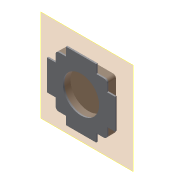
# Autodesk Inventor part: 30_Cube_counterplate_LEDmount
Saved by Autodesk Inventor 2019.4 (Build 234330000, 330)
## iProperties
Created: 2021-05-03
Part Number: 30_Cube_counterplate_LEDmount
Material: Generic
Document SubType Name: Modeling
Designer: diederichbenedict
Density: 1 g/cm^3
Appearance: Default
Author: diederichbenedict
Autodesk Inventor part; units mm, degrees
ref_plane "YZ Plane" through (0, 0, 0) normal (1, 0, 0) x (0, 1, 0)
ref_plane "XZ Plane" through (0, 0, 0) normal (0, 1, 0) x (-1, 0, 0)
ref_plane "XY Plane" through (0, 0, 0) normal (0, 0, 1) x (1, 0, 0)
ref_plane "Work Plane1" through (15.4052, 15.0652, 4.9) normal (0, 0, 1) x (0, 1, 0)
sketch "Sketch1" plane through (15.4052, 15.0652, 4.9) normal (0, 0, 1) x (0, 1, 0)
  circle A0 centre (5.7948, 15.4052) radius 2.5 projected
  circle A1 centre (-15.6052, -5.7948) radius 2.5 projected
  line L0 (-20.0856, 39.0762) -> (-20.0856, 40.2052) projected
  line L1 (-20.0856, 40.2052) -> (-38.2052, 40.2052) projected
  arc A2 (-38.2052, 40.2052) -> (-40.2052, 38.2052) centre (-38.2052, 38.2052) ccw projected
  line L2 (-40.2052, 20.2953) -> (-40.2052, 38.2052) projected
  line L3 (-40.2052, 20.2953) -> (-39.0783, 20.2953) projected
  arc A3 (-39.0783, 20.2953) -> (-38.6768, 20.6232) centre (-39.0783, 20.7051) ccw projected
  arc A4 (-34.5391, 20.2052) -> (-38.6768, 20.6232) centre (-36.6291, 20.2052) ccw projected
  line L4 (-34.5391, 20.2052) -> (-34.5391, 10.4067) projected
  arc A5 (-38.647, 9.8643) -> (-34.5391, 10.4067) centre (-36.6023, 10.2052) ccw projected
  line L5 (-38.647, 9.8643) -> (-38.6775, 9.9849) projected
  arc A6 (-38.6775, 9.9849) -> (-39.0762, 10.3249) centre (-39.083, 9.9131) ccw projected
  line L6 (-39.0762, 10.3249) -> (-40.2052, 10.3249) projected
  line L7 (-40.2052, -7.7948) -> (-40.2052, 10.3249) projected
  arc A7 (-40.2052, -7.7948) -> (-38.2052, -9.7948) centre (-38.2052, -7.7948) ccw projected
  line L8 (-38.2052, -9.7948) -> (-20.2052, -9.7948) projected
  line L9 (-20.2052, -9.7948) -> (-20.2052, -10.8453) projected
  arc A8 (-20.6052, -11.3352) -> (-20.2052, -10.8453) centre (-20.7052, -10.8453) ccw projected
  arc A9 (-20.6052, -11.3352) -> (-20.2052, -15.2948) centre (-20.2052, -13.2948) ccw projected
  line L10 (-20.2052, -15.2948) -> (-10.2052, -15.2948) projected
  arc A10 (-10.2052, -15.2948) -> (-9.8052, -11.3352) centre (-10.2052, -13.2948) ccw projected
  arc A11 (-10.2052, -10.8453) -> (-9.8052, -11.3352) centre (-9.7052, -10.8453) ccw projected
  line L11 (-10.2052, -10.8453) -> (-10.2052, -9.7948) projected
  line L12 (-10.2052, -9.7948) -> (7.7948, -9.7948) projected
  arc A12 (7.7948, -9.7948) -> (9.7948, -7.7948) centre (7.7948, -7.7948) ccw projected
  line L13 (9.7948, 10.2052) -> (9.7948, -7.7948) projected
  line L14 (9.7948, 10.2052) -> (10.8453, 10.2052) projected
  arc A13 (11.3352, 9.8052) -> (10.8453, 10.2052) centre (10.8453, 9.7052) ccw projected
  arc A14 (11.3352, 9.8052) -> (15.2948, 10.2052) centre (13.2948, 10.2052) ccw projected
  line L15 (15.2948, 10.2052) -> (15.2948, 20.2052) projected
  arc A15 (15.2948, 20.2052) -> (11.3352, 20.6052) centre (13.2948, 20.2052) ccw projected
  arc A16 (10.8453, 20.2052) -> (11.3352, 20.6052) centre (10.8453, 20.7052) ccw projected
  line L16 (10.8453, 20.2052) -> (9.7948, 20.2052) projected
  line L17 (9.7948, 38.2052) -> (9.7948, 20.2052) projected
  arc A17 (9.7948, 38.2052) -> (7.7948, 40.2052) centre (7.7948, 38.2052) ccw projected
  line L18 (7.7948, 40.2052) -> (-10.1151, 40.2052) projected
  line L19 (-10.1151, 40.2052) -> (-10.1151, 39.0783) projected
  arc A18 (-10.1151, 39.0783) -> (-9.7873, 38.6768) centre (-9.7054, 39.0783) ccw projected
  arc A19 (-10.2052, 34.5391) -> (-9.7873, 38.6768) centre (-10.2052, 36.6291) ccw projected
  line L20 (-10.2052, 34.5391) -> (-20.0038, 34.5391) projected
  arc A20 (-20.5462, 38.647) -> (-20.0038, 34.5391) centre (-20.2052, 36.6023) ccw projected
  line L21 (-20.5462, 38.647) -> (-20.4256, 38.6775) projected
  arc A21 (-20.4256, 38.6775) -> (-20.0856, 39.0762) centre (-20.4974, 39.083) ccw projected
  line L22 (-0.2052, 32.2052) -> (-30.2052, 32.2052) projected
  arc A22 (1.7948, 30.2052) -> (-0.2052, 32.2052) centre (-0.2052, 30.2052) ccw projected
  line L23 (1.7948, 30.2052) -> (1.7948, 0.2052) projected
  arc A23 (-0.2052, -1.7948) -> (1.7948, 0.2052) centre (-0.2052, 0.2052) ccw projected
  line L24 (-0.2052, -1.7948) -> (-30.2052, -1.7948) projected
  arc A24 (-32.2052, 0.2052) -> (-30.2052, -1.7948) centre (-30.2052, 0.2052) ccw projected
  line L25 (-32.2052, 0.2052) -> (-32.2052, 30.2052) projected
  arc A25 (-30.2052, 32.2052) -> (-32.2052, 30.2052) centre (-30.2052, 30.2052) ccw projected
  circle A26 centre (-35.2052, 35.2052) radius 2.425 projected
  circle A27 centre (-29.7052, 36.0052) radius 2.65 projected
  circle A28 centre (-36.0052, 29.7052) radius 2.65 projected
  circle A29 centre (-35.2052, -4.7948) radius 2.425 projected
  circle A30 centre (-29.7052, -5.5948) radius 2.65 projected
  circle A31 centre (-36.0052, 0.7052) radius 2.65 projected
  circle A32 centre (4.7948, 35.2052) radius 2.425 projected
  circle A33 centre (-0.7052, 36.0052) radius 2.65 projected
  circle A34 centre (5.5948, 29.7052) radius 2.65 projected
  circle A35 centre (5.5948, 0.7052) radius 2.65 projected
  circle A36 centre (-0.7052, -5.5948) radius 2.65 projected
  circle A37 centre (4.7948, -4.7948) radius 2.425 projected
  point P0 (-15.0652, 15.4052)
extrude "Extrusion1" add sketch "Sketch1" against normal blind 5 draft -1 contours A22 L23 A23 L24 A24 L25 A25 L22
sketch "Sketch2" plane through (15.4052, 15.0652, 4.9) normal (0, 0, 1) x (1, 0, 0)
  circle A0 centre (-26.2552, -7.0652) radius 3 projected
  circle A1 centre (-26.2552, -23.0652) radius 3 projected
  circle A2 centre (-4.2552, -15.0652) radius 1.6 projected
  line L0 (-50.1952, -15.0652) -> (19.3848, -15.0652)
  circle A3 centre (-15.4052, -15.0652) radius 12
  dimension "d4" = 24
  constraints: 2 end point, 1 centre point, 1 coincident, 1 horizontal, 2 other
  measures "d4" diameter of A3
extrude "Extrusion2" cut sketch "Sketch2" against normal blind 4 contours A0 A3 | A0 A3 A2 L0 | A3 L0 A2 | L0 A2 A3 A1 | L0 A3 A2 | A1 A3 picked at (-24.6691, -8.292) picked at (-4.1694, -14.672) picked at (-4.1694, -15.4584) picked at (-24.6691, -21.8384)
sketch "Sketch4" plane through (15.4052, 15.0652, 4.9) normal (0, 0, 1) x (1, 0, 0)
  circle A0 centre (-15.4052, -15.0652) radius 12 construction
  line L0 (-32.2052, -0.2052) -> (-32.2052, -30.2052) construction
  arc A1 (-32.2052, -30.2052) -> (-30.2052, -32.2052) centre (-30.2052, -30.2052) ccw construction
  line L1 (-30.2052, -32.2052) -> (-0.2052, -32.2052) construction
  arc A2 (-0.2052, -32.2052) -> (1.7948, -30.2052) centre (-0.2052, -30.2052) ccw construction
  line L2 (1.7948, -30.2052) -> (1.7948, -0.2052) construction
  arc A3 (1.7948, -0.2052) -> (-0.2052, 1.7948) centre (-0.2052, -0.2052) ccw construction
  line L3 (-0.2052, 1.7948) -> (-30.2052, 1.7948) construction
  arc A4 (-30.2052, 1.7948) -> (-32.2052, -0.2052) centre (-30.2052, -0.2052) ccw construction
  line L4 (-37.9052, -25.0652) -> (7.0948, -25.0652) construction
  line L5 (7.0948, -25.0652) -> (7.0948, -5.0652) construction
  line L6 (7.0948, -5.0652) -> (-37.9052, -5.0652) construction
  line L7 (-37.9052, -5.0652) -> (-37.9052, -25.0652) construction
  line L8 (-37.9052, -25.0652) -> (7.0948, -5.0652) construction
  line L9 (7.0948, -25.0652) -> (-37.9052, -5.0652) construction
  line L10 (-25.4052, 7.4348) -> (-5.4052, 7.4348) construction
  line L11 (-5.4052, 7.4348) -> (-5.4052, -37.5652) construction
  line L12 (-5.4052, -37.5652) -> (-25.4052, -37.5652) construction
  line L13 (-25.4052, -37.5652) -> (-25.4052, 7.4348) construction
  line L14 (-25.4052, 7.4348) -> (-5.4052, -37.5652) construction
  line L15 (-5.4052, 7.4348) -> (-25.4052, -37.5652) construction
  line L16 (1.7075, -30.2052) -> (1.7075, -0.2052) construction
  line L17 (-30.2052, -32.2052) -> (-0.2052, -32.2052) construction
  line L18 (-32.118, -0.2052) -> (-32.118, -30.2052) construction
  line L19 (-0.2052, 1.7948) -> (-30.2052, 1.7948) construction
  line L20 (7.0948, -5.0652) -> (1.7075, -5.0652)
  line L21 (1.7075, -5.0652) -> (1.7075, -25.0652)
  line L22 (1.7075, -25.0652) -> (7.0948, -25.0652)
  line L23 (7.0948, -25.0652) -> (7.0948, -5.0652)
  line L24 (-5.4052, -37.5652) -> (-25.4052, -37.5652)
  line L25 (-25.4052, -37.5652) -> (-25.4052, -32.2052)
  line L26 (-25.4052, -32.2052) -> (-5.4052, -32.2052)
  line L27 (-5.4052, -32.2052) -> (-5.4052, -37.5652)
  line L28 (-32.2052, -25.0652) -> (-37.9052, -25.0652)
  line L29 (-37.9052, -25.0652) -> (-37.9052, -5.0652)
  line L30 (-37.9052, -5.0652) -> (-32.2052, -5.0652)
  line L31 (-32.2052, -5.0652) -> (-32.2052, -25.0652)
  line L32 (-25.4052, 1.7948) -> (-5.4052, 1.7948)
  line L33 (-5.4052, 1.7948) -> (-5.4052, 7.4348)
  line L34 (-5.4052, 7.4348) -> (-25.4052, 7.4348)
  line L35 (-25.4052, 7.4348) -> (-25.4052, 1.7948)
  point P0 (1.7948, -5.0652)
  point P1 (-5.4052, -32.2052)
  point P2 (-32.118, -5.0652)
  point P3 (-5.4052, 1.7948)
  dimension "d7" = 45
  dimension "d8" = 20
  dimension "d9" = 20
  dimension "d10" = 45
  constraints: 56 end point, 16 point on line, 12 parallel, 6 horizontal, 6 perpendicular, 4 midpoint
  measures "d7" distance of L6.end L5.end
  measures "d8" distance of L5.end L4.end
  measures "d9" distance of L11.end L12.end
  measures "d10" distance of L10.end L11.end
extrude "Extrusion4" add sketch "Sketch4" along normal blind 1
sketch "Sketch5" plane through (15.4052, 15.0652, 4.9) normal (0, 0, 1) x (1, 0, 0)
  line L0 (1.7075, -5.0652) -> (1.7948, -5.0652) projected
  line L1 (1.7948, -5.0652) -> (1.7948, -0.2052) projected
  arc A0 (1.7948, -0.2052) -> (-0.2052, 1.7948) centre (-0.2052, -0.2052) ccw projected
  line L2 (-0.2052, 1.7948) -> (-5.4052, 1.7948) projected
  line L3 (-5.4052, 1.7948) -> (-25.4052, 1.7948) projected
  line L4 (-25.4052, 1.7948) -> (-30.2052, 1.7948) projected
  arc A1 (-30.2052, 1.7948) -> (-32.2052, -0.2052) centre (-30.2052, -0.2052) ccw projected
  line L5 (-32.2052, -0.2052) -> (-32.2052, -5.0652) projected
  line L6 (-32.2052, -5.0652) -> (-32.2052, -25.0652) projected
  line L7 (-32.2052, -25.0652) -> (-32.2052, -30.2052) projected
  arc A2 (-32.2052, -30.2052) -> (-30.2052, -32.2052) centre (-30.2052, -30.2052) ccw projected
  line L8 (-30.2052, -32.2052) -> (-25.4052, -32.2052) projected
  line L9 (-25.4052, -32.2052) -> (-5.4052, -32.2052) projected
  line L10 (-5.4052, -32.2052) -> (-0.2052, -32.2052) projected
  arc A3 (-0.2052, -32.2052) -> (1.7948, -30.2052) centre (-0.2052, -30.2052) ccw projected
  line L11 (1.7948, -30.2052) -> (1.7948, -25.0652) projected
  line L12 (1.7948, -25.0652) -> (1.7075, -25.0652) projected
  line L13 (1.7075, -25.0652) -> (1.7075, -5.0652) projected
  circle A4 centre (-15.4052, -15.0652) radius 12 projected
extrude "Extrusion5" add sketch "Sketch5" along normal blind 1
body "Solid1"
